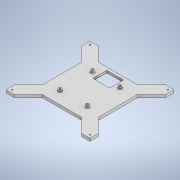
# Autodesk Inventor part: pi_base
Saved by Autodesk Inventor 2021.3 (Build 253353010, 353A)
## iProperties
Created: 2021-10-20
Part Number: pi_base
Material: Generic
Document SubType Name: Modeling
Designer: jesse
Density: 1 g/cm^3
Appearance: Default
Author: jesse
Autodesk Inventor part; units mm, degrees
ref_plane "YZ Plane" through (0, 0, 0) normal (1, 0, 0) x (0, 1, 0)
ref_plane "XZ Plane" through (0, 0, 0) normal (0, 1, 0) x (-1, 0, 0)
ref_plane "XY Plane" through (0, 0, 0) normal (0, 0, 1) x (1, 0, 0)
sketch "Sketch1" plane through (0, 0, 0) normal (0, 1, 0) x (-1, 0, 0)
  line L0 (80.0781, 66.9922) -> (-69.9219, 66.9922)
  line L1 (-69.9219, 66.9922) -> (-69.9219, -83.0078)
  line L2 (-69.9219, -83.0078) -> (80.0781, -83.0078)
  line L3 (80.0781, -83.0078) -> (80.0781, 66.9922)
  circle A0 centre (74.5781, -77.5078) radius 1.3
  line L4 (80.0781, -8.0078) -> (-69.9219, -8.0078)
  line L5 (5.0781, -83.0078) -> (5.0781, 66.9922)
  circle A1 centre (-64.4219, -77.5078) radius 1.3
  line L6 (-69.9219, -8.0078) -> (80.0781, -8.0078)
  circle A2 centre (74.5781, 61.4922) radius 1.3
  circle A3 centre (-64.4219, 61.4922) radius 1.3
  point P0 (0, 0)
  dimension "d0" = 150
  dimension "d1" = 150
  dimension "d4" = 2.6
  dimension "d8" = 5.5
  dimension "d9" = 5.5
  constraints: 14 end point, 5 symmetric about line, 4 centre point, 4 midpoint, 2 parallel, 1 horizontal, 1 perpendicular, 3 other
  measures "d0" distance of L2.end L0.start
  measures "d1" distance of L1.end L2.end
  measures "d4" diameter of A0
  measures "d8" distance from line of L2 A0.centre
  measures "d9" distance from line of L3 A0.centre
extrude "Extrusion1" add sketch "Sketch1" along normal blind 5
sketch "Sketch2" plane through (0, 5, 0) normal (0, 1, 0) x (1, 0, 0)
  line L0 (-29.5781, 37.0078) -> (19.4219, 37.0078)
  line L1 (19.4219, 37.0078) -> (19.4219, -20.9922)
  line L2 (19.4219, -20.9922) -> (-29.5781, -20.9922)
  line L3 (-29.5781, -20.9922) -> (-29.5781, 37.0078)
  line L4 (-5.0781, 37.0078) -> (-5.0781, -20.9922)
  line L5 (19.4219, 8.0078) -> (-29.5781, 8.0078)
  line L6 (69.9219, 83.0078) -> (-80.0781, 83.0078) projected
  line L7 (69.9219, -66.9922) -> (69.9219, 83.0078) projected
  circle A0 centre (-29.5781, 37.0078) radius 1.3
  circle A1 centre (19.4219, 37.0078) radius 1.3
  circle A2 centre (-29.5781, -20.9922) radius 1.3
  circle A3 centre (19.4219, -20.9922) radius 1.3
  line L8 (-80.0781, 83.0078) -> (-80.0781, -66.9922) projected
  line L9 (-80.0781, 68.0078) -> (-55.0781, 43.0078)
  line L10 (-55.0781, 43.0078) -> (-55.0781, -26.9922)
  line L11 (-55.0781, -26.9922) -> (-80.0781, -51.9922)
  line L12 (-80.0781, -66.9922) -> (69.9219, -66.9922) projected
  line L13 (69.9219, 68.0078) -> (44.9219, 43.0078)
  line L14 (44.9219, 43.0078) -> (44.9219, -26.9922)
  line L15 (44.9219, -26.9922) -> (69.9219, -51.9922)
  line L16 (-65.0781, 83.0078) -> (-40.0781, 58.0078)
  line L17 (-40.0781, 58.0078) -> (29.9219, 58.0078)
  line L18 (29.9219, 58.0078) -> (54.9219, 83.0078)
  line L19 (-65.0781, -66.9922) -> (-40.0781, -41.9922)
  line L20 (-40.0781, -41.9922) -> (29.9219, -41.9922)
  line L21 (29.9219, -41.9922) -> (54.9219, -66.9922)
  point P0 (0, 0)
  dimension "d10" = 58
  dimension "d11" = 49
  dimension "d12" = 75
  dimension "d13" = 75
  dimension "d14" = 2.6
  dimension "d15" = 2.6
  dimension "d16" = 2.6
  dimension "d17" = 2.6
  dimension "d18" = 15
  dimension "d19" = 15
  dimension "d20" = 25
  dimension "d21" = 25
  dimension "d22" = 25
  dimension "d23" = 25
  dimension "d24" = 25
  constraints: 36 end point, 6 point on line, 4 centre point, 4 coincident, 4 midpoint, 4 symmetric about line, 2 horizontal, 2 parallel, 2 perpendicular
  measures "d10" distance of L0.end L1.end
  measures "d11" distance of L0.start L0.end
  measures "d12" distance between parallel lines of L6 L5
  measures "d13" distance between parallel lines of L7 L4
  measures "d14" diameter of A0
  measures "d15" diameter of A1
  measures "d16" diameter of A2
  measures "d17" diameter of A3
  measures "d18" distance from line of L6 L9.start
  measures "d19" distance from line of L12 L11.end
  measures "d20" distance from line of L8 L9.end
  measures "d21" distance from line of L8 L10.end
  measures "d22" horizontal distance of L9.start L9.end
  measures "d23" horizontal distance of L11.end L10.end
  measures "d24" horizontal distance of L17.end L18.end
extrude "Extrusion2" cut sketch "Sketch2" against normal through all contours L3 A0 L0 | L0 A0 L3 | A1 L1 L0 | L0 L1 A1 | A2 L2 L3 | L3 L2 A2 | A3 L1 L2 | L2 L1 A3 | L18 L17 L16 L6 | L7 L15 L14 L13 | L9 L10 L11 L8 | L12 L19 L20 L21
sketch "Sketch3" plane through (0, 5, 0) normal (0, 1, 0) x (1, 0, 0)
  line L0 (-20.0781, 53.0078) -> (9.9219, 53.0078)
  line L1 (9.9219, 53.0078) -> (9.9219, 28.0078)
  line L2 (9.9219, 28.0078) -> (-20.0781, 28.0078)
  line L3 (-20.0781, 28.0078) -> (-20.0781, 53.0078)
  line L4 (29.9219, 58.0078) -> (-40.0781, 58.0078) projected
  line L5 (-5.0781, 53.0078) -> (-5.0781, 28.0078)
  line L6 (44.9219, -26.9922) -> (44.9219, 43.0078) projected
  point P0 (0, 0)
  dimension "d27" = 30
  dimension "d28" = 25
  dimension "d29" = 5
  dimension "d44" = 50
  constraints: 10 end point, 2 midpoint, 2 parallel, 1 horizontal, 1 perpendicular
  measures "d27" distance between parallel lines of L1 L3
  measures "d28" distance of L0.end L1.end
  measures "d29" distance between parallel lines of L0 L4
  measures "d44" distance between parallel lines of L6 L5
extrude "Extrusion3" cut sketch "Sketch3" against normal through all
fillet "Fillet1" radius 1 8 edges at (-20.0781, 2.5, -28.0078) (-20.0781, 0, -40.5078) (-5.0781, 0, -28.0078) (9.9219, 0, -40.5078) (-5.0781, 0, -53.0078) (9.9219, 2.5, -53.0078) (9.9219, 2.5, -28.0078) (-20.0781, 2.5, -53.0078)
sketch "Sketch4" plane through (0, 5, 0) normal (0, 1, 0) x (1, 0, 0)
  circle A0 centre (-29.5781, 37.0078) radius 2.8
  circle A1 centre (19.4219, 37.0078) radius 2.8
  circle A2 centre (19.4219, -20.9922) radius 2.8
  circle A3 centre (-29.5781, -20.9922) radius 2.8
  circle A4 centre (-29.5781, 37.0078) radius 1.3
  circle A5 centre (19.4219, 37.0078) radius 1.3
  circle A6 centre (19.4219, -20.9922) radius 1.3
  circle A7 centre (-29.5781, -20.9922) radius 1.3
  point P0 (0, 0)
  dimension "d33" = 5.6
  dimension "d34" = 5.6
  dimension "d35" = 5.6
  dimension "d36" = 5.6
  constraints: 8 centre point, 6 coincident
  measures "d33" diameter of A3
  measures "d34" diameter of A2
  measures "d35" diameter of A1
  measures "d36" diameter of A0
extrude "Extrusion4" add sketch "Sketch4" along normal blind 4 contours A0 | A1 | A2 | A3 | A4 | A5 | A6 | A7
sketch "Sketch5" plane through (-29.5781, 9, -37.0078) normal (0, 1, 0) x (1, 0, 0)
  circle A0 centre (0, 0) radius 1.3 projected
  circle A1 centre (0, 0) radius 1.3
  circle A2 centre (49, 0) radius 1.3 projected
  circle A3 centre (49, 0) radius 1.3
  circle A4 centre (49, -58) radius 1.3 projected
  circle A5 centre (49, -58) radius 1.3
  circle A6 centre (0, -58) radius 1.3 projected
  circle A7 centre (0, -58) radius 1.3
  point P0 (29.5781, -37.0078)
  constraints: 4 centre point, 4 coincident
extrude "Extrusion5" cut sketch "Sketch5" against normal through all
fillet "Fillet2" radius 1 4 edges at (-32.3781, 5, -37.0078) (-32.3781, 5, 20.9922) (16.6219, 5, 20.9922) (16.6219, 5, -37.0078)
fillet "Fillet3" radius 1 4 edges at (-80.0781, 2.5, 66.9922) (-80.0781, 2.5, -83.0078) (69.9219, 2.5, 66.9922) (69.9219, 2.5, -83.0078)
body "Solid1"
